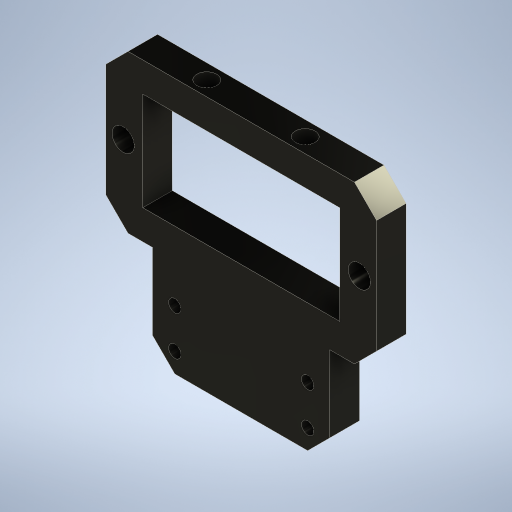
# Autodesk Inventor part: ServoCarrier
Saved by Autodesk Inventor 2024.3 (Build 283343000, 343)
## iProperties
Created: 2025-01-07
Part Number: ServoCarrier
Material: Generic
Document SubType Name: Modeling
Designer: migue
Density: 1 g/cm^3
Appearance: Gunmetal
Author: migue
Autodesk Inventor part; units mm, degrees
ref_plane "YZ Plane" through (0, 0, 0) normal (1, 0, 0) x (0, 1, 0)
ref_plane "XZ Plane" through (0, 0, 0) normal (0, 1, 0) x (-1, 0, 0)
ref_plane "XY Plane" through (0, 0, 0) normal (0, 0, 1) x (1, 0, 0)
sketch "Sketch1" plane through (0, 0, 0) normal (0, 0, 1) x (1, 0, 0)
  line L0 (-20, 10) -> (20, 10)
  line L1 (20, 10) -> (20, -10)
  line L2 (20, -10) -> (-20, -10)
  line L3 (-20, -10) -> (-20, 10)
  line L4 (-20, 10) -> (20, -10) construction
  line L5 (20, 10) -> (-20, -10) construction
  line L6 (-27.5, 16) -> (27.5, 16)
  line L7 (27.5, 16) -> (27.5, -16)
  line L8 (27.5, -16) -> (-27.5, -16)
  line L9 (-27.5, -16) -> (-27.5, 16)
  line L10 (-27.5, 16) -> (27.5, -16) construction
  line L11 (27.5, 16) -> (-27.5, -16) construction
  line L12 (0, 0) -> (0, 16) construction
  circle A0 centre (-24, 0) radius 2.25
  circle A1 centre (24, 0) radius 2.25
  dimension "d0" = 40
  dimension "d1" = 20
  dimension "d2" = 32
  dimension "d3" = 55
  dimension "d4" = 4.5
  dimension "d5" = 24
  constraints: 26 end point, 5 midpoint, 4 parallel, 2 centre point, 2 horizontal, 2 perpendicular, 1 symmetric about line, 1 other
  measures "d0" distance of L0.start L0.end
  measures "d1" distance of L0.end L1.end
  measures "d2" distance of L6.end L7.end
  measures "d3" distance of L6.start L6.end
  measures "d4" diameter of A0
  measures "d5" distance of A0.centre L12.start
extrude "Extrusion1" add sketch "Sketch1" along normal blind 6
chamfer "Chamfer1" distance 4.5 angle 45 4 edges at (27.5, 16, 3) (27.5, -16, 3) (-27.5, -16, 3) (-27.5, 16, 3)
sketch "Sketch2" plane through (-23, 16, 0) normal (0, 1, 0) x (1, 0, 0)
  line L0 (50.5, -6) -> (50.5, 0) projected
  line L1 (50.5, -3) -> (-4.5, -3) construction
  line L2 (-4.5, 0) -> (-4.5, -6) projected
  line L3 (23, 0) -> (23, -6) construction
  circle A0 centre (33, -3) radius 2
  circle A1 centre (13, -3) radius 2
  dimension "d11" = 10
  dimension "d12" = 4
  constraints: 4 end point, 2 centre point, 2 midpoint, 1 point on line, 1 symmetric about line, 1 vertical, 1 other
  measures "d11" distance from line of A0.centre L3
  measures "d12" diameter of A0
extrude "Extrusion2" cut sketch "Sketch2" against normal blind 15
sketch "Sketch3" plane through (0, 0, 6) normal (0, 0, 1) x (1, 0, 0)
  line L0 (-23, -16) -> (23, -16) projected
  line L1 (0, -16) -> (-18, -16)
  line L2 (-18, -16) -> (-18, -36)
  line L3 (-18, -36) -> (0, -36)
  line L4 (0, -36) -> (0, -16)
  circle A0 centre (-13.5, -24) radius 1.25
  line L5 (-13.5, -24) -> (-13.5, -32) construction
  circle A1 centre (-13.5, -32) radius 1.25
  line L6 (23, -16) -> (-23, -16)
  line L7 (18, -16) -> (18, -36)
  line L8 (18, -36) -> (0, -36)
  circle A2 centre (13.5, -24) radius 1.25
  circle A3 centre (13.5, -32) radius 1.25
  line L9 (-27.5, 11.5) -> (-27.5, -11.5) projected
  point P0 (0, 0)
  dimension "d17" = 18
  dimension "d18" = 20
  dimension "d19" = 2.5
  dimension "d20" = 2.5
  dimension "d21" = 8
  dimension "d22" = 16
  dimension "d26" = 13.5
  constraints: 16 end point, 6 symmetric about line, 4 centre point, 2 parallel, 1 coincident, 1 horizontal, 1 midpoint, 1 perpendicular, 1 vertical, 2 other
  measures "d17" distance of L3.end L2.end
  measures "d18" distance of L2.end L1.end
  measures "d19" diameter of A0
  measures "d20" diameter of A1
  measures "d21" distance of L5.start L5.end
  measures "d22" distance from line of L0 L5.end
  measures "d26" distance from line of A2.centre L4
extrude "Extrusion3" add sketch "Sketch3" against normal blind 6
chamfer "Chamfer2" distance 4.5 angle 45 2 edges at (18, -36, 3) (-18, -36, 3)
body "Solid1"
